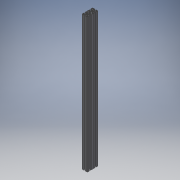
# Autodesk Inventor part: PERFIL_ESTRUTURAL_40X80_EIXO_Y
Saved by Autodesk Inventor 2018 (Build 220112000, 112)
## iProperties
Created: 2018-10-08
Part Number: PERFIL_ESTRUTURAL_40X80_EIXO_Y
Material: Genérico
Document SubType Name: Modeling
Designer: Georgines
Density: 1 g/cm^3
Appearance: Padrão
Author: Georgines
Autodesk Inventor part; units mm, degrees
ref_plane "YZ Plane" through (0, 0, 0) normal (1, 0, 0) x (0, 1, 0)
ref_plane "XZ Plane" through (0, 0, 0) normal (0, 1, 0) x (-1, 0, 0)
ref_plane "XY Plane" through (0, 0, 0) normal (0, 0, 1) x (1, 0, 0)
sketch "Esboço1" plane through (0, 0, 0) normal (0, 0, 1) x (1, 0, 0)
  line L0 (4.1513, 39.5067) -> (4.1513, 35.6766)
  arc A0 (4.3212, 39.6766) -> (4.1513, 39.5067) centre (4.3212, 39.5067) ccw
  line L1 (11.1013, 39.6766) -> (4.3212, 39.6766)
  line L2 (11.1013, 39.4266) -> (11.1013, 39.6766)
  line L3 (13.1013, 39.4266) -> (11.1013, 39.4266)
  line L4 (13.1013, 39.6766) -> (13.1013, 39.4266)
  line L5 (18.6013, 39.6766) -> (13.1013, 39.6766)
  arc A1 (20.1013, 38.1766) -> (18.6013, 39.6766) centre (18.6013, 38.1766) ccw
  line L6 (20.1013, 32.6766) -> (20.1013, 38.1766)
  line L7 (19.8513, 32.6766) -> (20.1013, 32.6766)
  line L8 (19.8513, 30.6766) -> (19.8513, 32.6766)
  line L9 (20.1013, 30.6766) -> (19.8513, 30.6766)
  line L10 (20.1013, 23.8965) -> (20.1013, 30.6766)
  arc A2 (19.9314, 23.7266) -> (20.1013, 23.8965) centre (19.9314, 23.8965) ccw
  line L11 (16.1013, 23.7266) -> (19.9314, 23.7266)
  line L12 (16.1013, 26.8766) -> (16.1013, 23.7266)
  line L13 (18.2013, 26.8766) -> (16.1013, 26.8766)
  line L14 (18.2013, 30.6766) -> (18.2013, 26.8766)
  line L15 (13.6368, 30.6766) -> (18.2013, 30.6766)
  arc A3 (13.6368, 30.6766) -> (12.9297, 30.3837) centre (13.6368, 29.6766) ccw
  line L16 (11.5658, 29.0197) -> (12.9297, 30.3837)
  arc A4 (11.5658, 29.0197) -> (10.1013, 25.4842) centre (15.1013, 25.4842) ccw
  line L17 (10.1013, 13.869) -> (10.1013, 25.4842)
  arc A5 (10.1013, 13.869) -> (11.5658, 10.3334) centre (15.1013, 13.869) ccw
  line L18 (12.9297, 8.9695) -> (11.5658, 10.3334)
  arc A6 (12.9297, 8.9695) -> (13.6368, 8.6766) centre (13.6368, 9.6766) ccw
  line L19 (18.2013, 8.6766) -> (13.6368, 8.6766)
  line L20 (18.2013, 12.4766) -> (18.2013, 8.6766)
  line L21 (16.1013, 12.4766) -> (18.2013, 12.4766)
  line L22 (16.1013, 15.6266) -> (16.1013, 12.4766)
  line L23 (19.9314, 15.6266) -> (16.1013, 15.6266)
  arc A7 (20.1013, 15.4567) -> (19.9314, 15.6266) centre (19.9314, 15.4567) ccw
  line L24 (20.1013, 8.6766) -> (20.1013, 15.4567)
  line L25 (19.8513, 8.6766) -> (20.1013, 8.6766)
  line L26 (19.8513, 6.6766) -> (19.8513, 8.6766)
  line L27 (20.1013, 6.6766) -> (19.8513, 6.6766)
  line L28 (20.1013, -7.3234) -> (20.1013, 6.6766)
  line L29 (19.8513, -7.3234) -> (20.1013, -7.3234)
  line L30 (19.8513, -9.3234) -> (19.8513, -7.3234)
  line L31 (20.1013, -9.3234) -> (19.8513, -9.3234)
  line L32 (20.1013, -16.1035) -> (20.1013, -9.3234)
  arc A8 (19.9314, -16.2734) -> (20.1013, -16.1035) centre (19.9314, -16.1035) ccw
  line L33 (16.1013, -16.2734) -> (19.9314, -16.2734)
  line L34 (16.1013, -13.1234) -> (16.1013, -16.2734)
  line L35 (18.2013, -13.1234) -> (16.1013, -13.1234)
  line L36 (18.2013, -9.3234) -> (18.2013, -13.1234)
  line L37 (13.6368, -9.3234) -> (18.2013, -9.3234)
  arc A9 (13.6368, -9.3234) -> (12.9297, -9.6163) centre (13.6368, -10.3234) ccw
  line L38 (11.5658, -10.9803) -> (12.9297, -9.6163)
  arc A10 (11.5658, -10.9803) -> (10.1013, -14.5158) centre (15.1013, -14.5158) ccw
  line L39 (10.1013, -26.131) -> (10.1013, -14.5158)
  arc A11 (10.1013, -26.131) -> (11.5658, -29.6666) centre (15.1013, -26.131) ccw
  line L40 (12.9297, -31.0305) -> (11.5658, -29.6666)
  arc A12 (12.9297, -31.0305) -> (13.6368, -31.3234) centre (13.6368, -30.3234) ccw
  line L41 (18.2013, -31.3234) -> (13.6368, -31.3234)
  line L42 (18.2013, -27.5234) -> (18.2013, -31.3234)
  line L43 (16.1013, -27.5234) -> (18.2013, -27.5234)
  line L44 (16.1013, -24.3734) -> (16.1013, -27.5234)
  line L45 (19.9314, -24.3734) -> (16.1013, -24.3734)
  arc A13 (20.1013, -24.5433) -> (19.9314, -24.3734) centre (19.9314, -24.5433) ccw
  line L46 (20.1013, -31.3234) -> (20.1013, -24.5433)
  line L47 (19.8513, -31.3234) -> (20.1013, -31.3234)
  line L48 (19.8513, -33.3234) -> (19.8513, -31.3234)
  line L49 (20.1013, -33.3234) -> (19.8513, -33.3234)
  line L50 (20.1013, -38.8234) -> (20.1013, -33.3234)
  arc A14 (18.6013, -40.3234) -> (20.1013, -38.8234) centre (18.6013, -38.8234) ccw
  line L51 (13.1013, -40.3234) -> (18.6013, -40.3234)
  line L52 (13.1013, -40.0734) -> (13.1013, -40.3234)
  line L53 (11.1013, -40.0734) -> (13.1013, -40.0734)
  line L54 (11.1013, -40.3234) -> (11.1013, -40.0734)
  line L55 (4.3212, -40.3234) -> (11.1013, -40.3234)
  arc A15 (4.1513, -40.1535) -> (4.3212, -40.3234) centre (4.3212, -40.1535) ccw
  line L56 (4.1513, -36.3234) -> (4.1513, -40.1535)
  line L57 (7.3013, -36.3234) -> (4.1513, -36.3234)
  line L58 (7.3013, -38.4234) -> (7.3013, -36.3234)
  line L59 (11.1013, -38.4234) -> (7.3013, -38.4234)
  line L60 (11.1013, -33.859) -> (11.1013, -38.4234)
  arc A16 (11.1013, -33.859) -> (10.8084, -33.1519) centre (10.1013, -33.859) ccw
  line L61 (9.4444, -31.7879) -> (10.8084, -33.1519)
  arc A17 (9.4444, -31.7879) -> (5.9089, -30.3234) centre (5.9089, -35.3234) ccw
  line L62 (-5.7063, -30.3234) -> (5.9089, -30.3234)
  arc A18 (-5.7063, -30.3234) -> (-9.2419, -31.7879) centre (-5.7063, -35.3234) ccw
  line L63 (-10.6058, -33.1519) -> (-9.2419, -31.7879)
  arc A19 (-10.6058, -33.1519) -> (-10.8987, -33.859) centre (-9.8987, -33.859) ccw
  line L64 (-10.8987, -38.4234) -> (-10.8987, -33.859)
  line L65 (-7.0987, -38.4234) -> (-10.8987, -38.4234)
  line L66 (-7.0987, -36.3234) -> (-7.0987, -38.4234)
  line L67 (-3.9487, -36.3234) -> (-7.0987, -36.3234)
  line L68 (-3.9487, -40.1535) -> (-3.9487, -36.3234)
  arc A20 (-4.1186, -40.3234) -> (-3.9487, -40.1535) centre (-4.1186, -40.1535) ccw
  line L69 (-10.8987, -40.3234) -> (-4.1186, -40.3234)
  line L70 (-10.8987, -40.0734) -> (-10.8987, -40.3234)
  line L71 (-12.8987, -40.0734) -> (-10.8987, -40.0734)
  line L72 (-12.8987, -40.3234) -> (-12.8987, -40.0734)
  line L73 (-18.3987, -40.3234) -> (-12.8987, -40.3234)
  arc A21 (-19.8987, -38.8234) -> (-18.3987, -40.3234) centre (-18.3987, -38.8234) ccw
  line L74 (-19.8987, -33.3234) -> (-19.8987, -38.8234)
  line L75 (-19.6487, -33.3234) -> (-19.8987, -33.3234)
  line L76 (-19.6487, -31.3234) -> (-19.6487, -33.3234)
  line L77 (-19.8987, -31.3234) -> (-19.6487, -31.3234)
  line L78 (-19.8987, -24.5433) -> (-19.8987, -31.3234)
  arc A22 (-19.7288, -24.3734) -> (-19.8987, -24.5433) centre (-19.7288, -24.5433) ccw
  line L79 (-15.8987, -24.3734) -> (-19.7288, -24.3734)
  line L80 (-15.8987, -27.5234) -> (-15.8987, -24.3734)
  line L81 (-17.9987, -27.5234) -> (-15.8987, -27.5234)
  line L82 (-17.9987, -31.3234) -> (-17.9987, -27.5234)
  line L83 (-13.4342, -31.3234) -> (-17.9987, -31.3234)
  arc A23 (-13.4342, -31.3234) -> (-12.7271, -31.0305) centre (-13.4342, -30.3234) ccw
  line L84 (-11.3632, -29.6666) -> (-12.7271, -31.0305)
  arc A24 (-11.3632, -29.6666) -> (-9.8987, -26.131) centre (-14.8987, -26.131) ccw
  line L85 (-9.8987, -14.5158) -> (-9.8987, -26.131)
  arc A25 (-9.8987, -14.5158) -> (-11.3632, -10.9803) centre (-14.8987, -14.5158) ccw
  line L86 (-12.7271, -9.6163) -> (-11.3632, -10.9803)
  arc A26 (-12.7271, -9.6163) -> (-13.4342, -9.3234) centre (-13.4342, -10.3234) ccw
  line L87 (-17.9987, -9.3234) -> (-13.4342, -9.3234)
  line L88 (-17.9987, -13.1234) -> (-17.9987, -9.3234)
  line L89 (-15.8987, -13.1234) -> (-17.9987, -13.1234)
  line L90 (-15.8987, -16.2734) -> (-15.8987, -13.1234)
  line L91 (-19.7288, -16.2734) -> (-15.8987, -16.2734)
  arc A27 (-19.8987, -16.1035) -> (-19.7288, -16.2734) centre (-19.7288, -16.1035) ccw
  line L92 (-19.8987, -9.3234) -> (-19.8987, -16.1035)
  line L93 (-19.6487, -9.3234) -> (-19.8987, -9.3234)
  line L94 (-19.6487, -7.3234) -> (-19.6487, -9.3234)
  line L95 (-19.8987, -7.3234) -> (-19.6487, -7.3234)
  line L96 (-19.8987, 6.6766) -> (-19.8987, -7.3234)
  line L97 (-19.6487, 6.6766) -> (-19.8987, 6.6766)
  line L98 (-19.6487, 8.6766) -> (-19.6487, 6.6766)
  line L99 (-19.8987, 8.6766) -> (-19.6487, 8.6766)
  line L100 (-19.8987, 15.4567) -> (-19.8987, 8.6766)
  arc A28 (-19.7288, 15.6266) -> (-19.8987, 15.4567) centre (-19.7288, 15.4567) ccw
  line L101 (-15.8987, 15.6266) -> (-19.7288, 15.6266)
  line L102 (-15.8987, 12.4766) -> (-15.8987, 15.6266)
  line L103 (-17.9987, 12.4766) -> (-15.8987, 12.4766)
  line L104 (-17.9987, 8.6766) -> (-17.9987, 12.4766)
  line L105 (-13.4342, 8.6766) -> (-17.9987, 8.6766)
  arc A29 (-13.4342, 8.6766) -> (-12.7271, 8.9695) centre (-13.4342, 9.6766) ccw
  line L106 (-11.3632, 10.3334) -> (-12.7271, 8.9695)
  arc A30 (-11.3632, 10.3334) -> (-9.8987, 13.869) centre (-14.8987, 13.869) ccw
  line L107 (-9.8987, 25.4842) -> (-9.8987, 13.869)
  arc A31 (-9.8987, 25.4842) -> (-11.3632, 29.0197) centre (-14.8987, 25.4842) ccw
  line L108 (-12.7271, 30.3837) -> (-11.3632, 29.0197)
  arc A32 (-12.7271, 30.3837) -> (-13.4342, 30.6766) centre (-13.4342, 29.6766) ccw
  line L109 (-17.9987, 30.6766) -> (-13.4342, 30.6766)
  line L110 (-17.9987, 26.8766) -> (-17.9987, 30.6766)
  line L111 (-15.8987, 26.8766) -> (-17.9987, 26.8766)
  line L112 (-15.8987, 23.7266) -> (-15.8987, 26.8766)
  line L113 (-19.7288, 23.7266) -> (-15.8987, 23.7266)
  arc A33 (-19.8987, 23.8965) -> (-19.7288, 23.7266) centre (-19.7288, 23.8965) ccw
  line L114 (-19.8987, 30.6766) -> (-19.8987, 23.8965)
  line L115 (-19.6487, 30.6766) -> (-19.8987, 30.6766)
  line L116 (-19.6487, 32.6766) -> (-19.6487, 30.6766)
  line L117 (-19.8987, 32.6766) -> (-19.6487, 32.6766)
  line L118 (-19.8987, 38.1766) -> (-19.8987, 32.6766)
  arc A34 (-18.3987, 39.6766) -> (-19.8987, 38.1766) centre (-18.3987, 38.1766) ccw
  line L119 (-12.8987, 39.6766) -> (-18.3987, 39.6766)
  line L120 (-12.8987, 39.4266) -> (-12.8987, 39.6766)
  line L121 (-10.8987, 39.4266) -> (-12.8987, 39.4266)
  line L122 (-10.8987, 39.6766) -> (-10.8987, 39.4266)
  line L123 (-4.1186, 39.6766) -> (-10.8987, 39.6766)
  arc A35 (-3.9487, 39.5067) -> (-4.1186, 39.6766) centre (-4.1186, 39.5067) ccw
  line L124 (-3.9487, 35.6766) -> (-3.9487, 39.5067)
  line L125 (-7.0987, 35.6766) -> (-3.9487, 35.6766)
  line L126 (-7.0987, 37.7766) -> (-7.0987, 35.6766)
  line L127 (-10.8987, 37.7766) -> (-7.0987, 37.7766)
  line L128 (-10.8987, 33.2121) -> (-10.8987, 37.7766)
  arc A36 (-10.8987, 33.2121) -> (-10.6058, 32.505) centre (-9.8987, 33.2121) ccw
  line L129 (-9.2419, 31.141) -> (-10.6058, 32.505)
  arc A37 (-9.2419, 31.141) -> (-5.7063, 29.6766) centre (-5.7063, 34.6766) ccw
  line L130 (5.9089, 29.6766) -> (-5.7063, 29.6766)
  arc A38 (5.9089, 29.6766) -> (9.4444, 31.141) centre (5.9089, 34.6766) ccw
  line L131 (10.8084, 32.505) -> (9.4444, 31.141)
  arc A39 (10.8084, 32.505) -> (11.1013, 33.2121) centre (10.1013, 33.2121) ccw
  line L132 (11.1013, 37.7766) -> (11.1013, 33.2121)
  line L133 (7.3013, 37.7766) -> (11.1013, 37.7766)
  line L134 (7.3013, 35.6766) -> (7.3013, 37.7766)
  line L135 (4.1513, 35.6766) -> (7.3013, 35.6766)
  arc A40 (0.9954, -13.532) -> (-0.7928, -13.532) centre (0.1013, -20.3234) ccw
  line L136 (-0.7928, -13.532) -> (-0.9429, -12.3919)
  arc A41 (-0.9429, -12.3919) -> (-2.9602, -12.9324) centre (0.1013, -20.3234) ccw
  line L137 (-2.9602, -12.9324) -> (-2.5201, -13.9949)
  arc A42 (-2.5201, -13.9949) -> (-3.9834, -14.8245) centre (0.1013, -20.3234) ccw
  line L138 (-3.9834, -14.8245) -> (-4.7102, -14.0977)
  arc A43 (-4.7688, -13.9563) -> (-4.7102, -14.0977) centre (-4.5688, -13.9563) ccw
  line L139 (-4.7688, -13.9563) -> (-4.7688, -12.4524)
  arc A44 (-4.7688, -12.4524) -> (-4.9688, -12.2524) centre (-4.9688, -12.4524) ccw
  line L140 (-4.9688, -12.2524) -> (-7.7698, -12.2524)
  arc A45 (-7.7698, -12.2524) -> (-7.9698, -12.4524) centre (-7.7698, -12.4524) ccw
  line L141 (-7.9698, -12.4524) -> (-7.9698, -15.2533)
  arc A46 (-7.9698, -15.2533) -> (-7.7698, -15.4533) centre (-7.7698, -15.2533) ccw
  line L142 (-7.7698, -15.4533) -> (-6.2659, -15.4533)
  arc A47 (-6.1244, -15.5119) -> (-6.2659, -15.4533) centre (-6.2659, -15.6533) ccw
  line L143 (-6.1244, -15.5119) -> (-5.3976, -16.2388)
  arc A48 (-5.3976, -16.2388) -> (-6.2273, -17.7021) centre (0.1013, -20.3234) ccw
  line L144 (-6.2273, -17.7021) -> (-7.2897, -17.262)
  arc A49 (-7.2897, -17.262) -> (-7.8303, -19.2792) centre (0.1013, -20.3234) ccw
  line L145 (-7.8303, -19.2792) -> (-6.6901, -19.4293)
  arc A50 (-6.6901, -19.4293) -> (-6.6901, -21.2175) centre (0.1013, -20.3234) ccw
  line L146 (-6.6901, -21.2175) -> (-7.8303, -21.3676)
  arc A51 (-7.8303, -21.3676) -> (-7.2897, -23.3849) centre (0.1013, -20.3234) ccw
  line L147 (-7.2897, -23.3849) -> (-6.2273, -22.9448)
  arc A52 (-6.2273, -22.9448) -> (-5.3976, -24.4081) centre (0.1013, -20.3234) ccw
  line L148 (-5.3976, -24.4081) -> (-6.1244, -25.1349)
  arc A53 (-6.2659, -25.1935) -> (-6.1244, -25.1349) centre (-6.2659, -24.9935) ccw
  line L149 (-6.2659, -25.1935) -> (-7.7698, -25.1935)
  arc A54 (-7.7698, -25.1935) -> (-7.9698, -25.3935) centre (-7.7698, -25.3935) ccw
  line L150 (-7.9698, -25.3935) -> (-7.9698, -28.1945)
  arc A55 (-7.9698, -28.1945) -> (-7.7698, -28.3945) centre (-7.7698, -28.1945) ccw
  line L151 (-7.7698, -28.3945) -> (-4.9688, -28.3945)
  arc A56 (-4.9688, -28.3945) -> (-4.7688, -28.1945) centre (-4.9688, -28.1945) ccw
  line L152 (-4.7688, -28.1945) -> (-4.7688, -26.6906)
  arc A57 (-4.7102, -26.5492) -> (-4.7688, -26.6906) centre (-4.5688, -26.6906) ccw
  line L153 (-4.7102, -26.5492) -> (-3.9834, -25.8223)
  arc A58 (-3.9834, -25.8223) -> (-2.5201, -26.652) centre (0.1013, -20.3234) ccw
  line L154 (-2.5201, -26.652) -> (-2.9602, -27.7145)
  arc A59 (-2.9602, -27.7145) -> (-0.9429, -28.255) centre (0.1013, -20.3234) ccw
  line L155 (-0.9429, -28.255) -> (-0.7928, -27.1148)
  arc A60 (-0.7928, -27.1148) -> (0.9954, -27.1148) centre (0.1013, -20.3234) ccw
  line L156 (0.9954, -27.1148) -> (1.1455, -28.255)
  arc A61 (1.1455, -28.255) -> (3.1628, -27.7145) centre (0.1013, -20.3234) ccw
  line L157 (3.1628, -27.7145) -> (2.7227, -26.652)
  arc A62 (2.7227, -26.652) -> (4.186, -25.8223) centre (0.1013, -20.3234) ccw
  line L158 (4.186, -25.8223) -> (4.9128, -26.5492)
  arc A63 (4.9714, -26.6906) -> (4.9128, -26.5492) centre (4.7714, -26.6906) ccw
  line L159 (4.9714, -26.6906) -> (4.9714, -28.1945)
  arc A64 (4.9714, -28.1945) -> (5.1714, -28.3945) centre (5.1714, -28.1945) ccw
  line L160 (5.1714, -28.3945) -> (7.9724, -28.3945)
  arc A65 (7.9724, -28.3945) -> (8.1724, -28.1945) centre (7.9724, -28.1945) ccw
  line L161 (8.1724, -28.1945) -> (8.1724, -25.3935)
  arc A66 (8.1724, -25.3935) -> (7.9724, -25.1935) centre (7.9724, -25.3935) ccw
  line L162 (7.9724, -25.1935) -> (6.4684, -25.1935)
  arc A67 (6.327, -25.1349) -> (6.4684, -25.1935) centre (6.4684, -24.9935) ccw
  line L163 (6.327, -25.1349) -> (5.6002, -24.4081)
  arc A68 (5.6002, -24.4081) -> (6.4299, -22.9448) centre (0.1013, -20.3234) ccw
  line L164 (6.4299, -22.9448) -> (7.4923, -23.3849)
  arc A69 (7.4923, -23.3849) -> (8.0328, -21.3676) centre (0.1013, -20.3234) ccw
  line L165 (8.0328, -21.3676) -> (6.8927, -21.2175)
  arc A70 (6.8927, -21.2175) -> (6.8927, -19.4293) centre (0.1013, -20.3234) ccw
  line L166 (6.8927, -19.4293) -> (8.0328, -19.2792)
  arc A71 (8.0328, -19.2792) -> (7.4923, -17.262) centre (0.1013, -20.3234) ccw
  line L167 (7.4923, -17.262) -> (6.4299, -17.7021)
  arc A72 (6.4299, -17.7021) -> (5.6002, -16.2388) centre (0.1013, -20.3234) ccw
  line L168 (5.6002, -16.2388) -> (6.327, -15.5119)
  arc A73 (6.4684, -15.4533) -> (6.327, -15.5119) centre (6.4684, -15.6533) ccw
  line L169 (6.4684, -15.4533) -> (7.9724, -15.4533)
  arc A74 (7.9724, -15.4533) -> (8.1724, -15.2533) centre (7.9724, -15.2533) ccw
  line L170 (8.1724, -15.2533) -> (8.1724, -12.4524)
  arc A75 (8.1724, -12.4524) -> (7.9724, -12.2524) centre (7.9724, -12.4524) ccw
  line L171 (7.9724, -12.2524) -> (5.1714, -12.2524)
  arc A76 (5.1714, -12.2524) -> (4.9714, -12.4524) centre (5.1714, -12.4524) ccw
  line L172 (4.9714, -12.4524) -> (4.9714, -13.9563)
  arc A77 (4.9128, -14.0977) -> (4.9714, -13.9563) centre (4.7714, -13.9563) ccw
  line L173 (4.9128, -14.0977) -> (4.186, -14.8245)
  arc A78 (4.186, -14.8245) -> (2.7227, -13.9949) centre (0.1013, -20.3234) ccw
  line L174 (2.7227, -13.9949) -> (3.1628, -12.9324)
  arc A79 (3.1628, -12.9324) -> (1.1455, -12.3919) centre (0.1013, -20.3234) ccw
  line L175 (1.1455, -12.3919) -> (0.9954, -13.532)
  arc A80 (-14.2427, -33.6068) -> (-16.5547, -33.6068) centre (-15.3987, -35.8234) ccw
  line L176 (-16.5547, -33.6068) -> (-16.8129, -33.3486)
  arc A81 (-16.8129, -33.3486) -> (-17.8736, -34.4092) centre (-17.3433, -33.8789) ccw
  line L177 (-17.8736, -34.4092) -> (-17.6154, -34.6674)
  arc A82 (-17.6154, -34.6674) -> (-17.6154, -36.9794) centre (-15.3987, -35.8234) ccw
  line L178 (-17.6154, -36.9794) -> (-17.8736, -37.2376)
  arc A83 (-17.8736, -37.2376) -> (-16.8129, -38.2983) centre (-17.3433, -37.768) ccw
  line L179 (-16.8129, -38.2983) -> (-16.5547, -38.0401)
  arc A84 (-16.5547, -38.0401) -> (-14.2427, -38.0401) centre (-15.3987, -35.8234) ccw
  line L180 (-14.2427, -38.0401) -> (-13.9845, -38.2983)
  arc A85 (-13.9845, -38.2983) -> (-12.9238, -37.2376) centre (-13.4542, -37.768) ccw
  line L181 (-12.9238, -37.2376) -> (-13.182, -36.9794)
  arc A86 (-13.182, -36.9794) -> (-13.182, -34.6674) centre (-15.3987, -35.8234) ccw
  line L182 (-13.182, -34.6674) -> (-12.9238, -34.4092)
  arc A87 (-12.9238, -34.4092) -> (-13.9845, -33.3486) centre (-13.4542, -33.8789) ccw
  line L183 (-13.9845, -33.3486) -> (-14.2427, -33.6068)
  arc A88 (14.4453, 32.9599) -> (16.7573, 32.9599) centre (15.6013, 35.1766) ccw
  line L184 (16.7573, 32.9599) -> (17.0155, 32.7017)
  arc A89 (17.0155, 32.7017) -> (18.0762, 33.7624) centre (17.5458, 33.232) ccw
  line L185 (18.0762, 33.7624) -> (17.818, 34.0206)
  arc A90 (17.818, 34.0206) -> (17.818, 36.3326) centre (15.6013, 35.1766) ccw
  line L186 (17.818, 36.3326) -> (18.0762, 36.5908)
  arc A91 (18.0762, 36.5908) -> (17.0155, 37.6514) centre (17.5458, 37.1211) ccw
  line L187 (17.0155, 37.6514) -> (16.7573, 37.3932)
  arc A92 (16.7573, 37.3932) -> (14.4453, 37.3932) centre (15.6013, 35.1766) ccw
  line L188 (14.4453, 37.3932) -> (14.1871, 37.6514)
  arc A93 (14.1871, 37.6514) -> (13.1264, 36.5908) centre (13.6567, 37.1211) ccw
  line L189 (13.1264, 36.5908) -> (13.3846, 36.3326)
  arc A94 (13.3846, 36.3326) -> (13.3846, 34.0206) centre (15.6013, 35.1766) ccw
  line L190 (13.3846, 34.0206) -> (13.1264, 33.7624)
  arc A95 (13.1264, 33.7624) -> (14.1871, 32.7017) centre (13.6567, 33.232) ccw
  line L191 (14.1871, 32.7017) -> (14.4453, 32.9599)
  arc A96 (-17.6154, 36.3326) -> (-17.6154, 34.0206) centre (-15.3987, 35.1766) ccw
  line L192 (-17.6154, 34.0206) -> (-17.8736, 33.7624)
  arc A97 (-17.8736, 33.7624) -> (-16.8129, 32.7017) centre (-17.3433, 33.232) ccw
  line L193 (-16.8129, 32.7017) -> (-16.5547, 32.9599)
  arc A98 (-16.5547, 32.9599) -> (-14.2427, 32.9599) centre (-15.3987, 35.1766) ccw
  line L194 (-14.2427, 32.9599) -> (-13.9845, 32.7017)
  arc A99 (-13.9845, 32.7017) -> (-12.9238, 33.7624) centre (-13.4542, 33.232) ccw
  line L195 (-12.9238, 33.7624) -> (-13.182, 34.0206)
  arc A100 (-13.182, 34.0206) -> (-13.182, 36.3326) centre (-15.3987, 35.1766) ccw
  line L196 (-13.182, 36.3326) -> (-12.9238, 36.5908)
  arc A101 (-12.9238, 36.5908) -> (-13.9845, 37.6514) centre (-13.4542, 37.1211) ccw
  line L197 (-13.9845, 37.6514) -> (-14.2427, 37.3932)
  arc A102 (-14.2427, 37.3932) -> (-16.5547, 37.3932) centre (-15.3987, 35.1766) ccw
  line L198 (-16.5547, 37.3932) -> (-16.8129, 37.6514)
  arc A103 (-16.8129, 37.6514) -> (-17.8736, 36.5908) centre (-17.3433, 37.1211) ccw
  line L199 (-17.8736, 36.5908) -> (-17.6154, 36.3326)
  arc A104 (14.4453, -38.0401) -> (16.7573, -38.0401) centre (15.6013, -35.8234) ccw
  line L200 (16.7573, -38.0401) -> (17.0155, -38.2983)
  arc A105 (17.0155, -38.2983) -> (18.0762, -37.2376) centre (17.5458, -37.768) ccw
  line L201 (18.0762, -37.2376) -> (17.818, -36.9794)
  arc A106 (17.818, -36.9794) -> (17.818, -34.6674) centre (15.6013, -35.8234) ccw
  line L202 (17.818, -34.6674) -> (18.0762, -34.4092)
  arc A107 (18.0762, -34.4092) -> (17.0155, -33.3486) centre (17.5458, -33.8789) ccw
  line L203 (17.0155, -33.3486) -> (16.7573, -33.6068)
  arc A108 (16.7573, -33.6068) -> (14.4453, -33.6068) centre (15.6013, -35.8234) ccw
  line L204 (14.4453, -33.6068) -> (14.1871, -33.3486)
  arc A109 (14.1871, -33.3486) -> (13.1264, -34.4092) centre (13.6567, -33.8789) ccw
  line L205 (13.1264, -34.4092) -> (13.3846, -34.6674)
  arc A110 (13.3846, -34.6674) -> (13.3846, -36.9794) centre (15.6013, -35.8234) ccw
  line L206 (13.3846, -36.9794) -> (13.1264, -37.2376)
  arc A111 (13.1264, -37.2376) -> (14.1871, -38.2983) centre (13.6567, -37.768) ccw
  line L207 (14.1871, -38.2983) -> (14.4453, -38.0401)
  arc A112 (6.4684, 24.5467) -> (6.327, 24.4881) centre (6.4684, 24.3467) ccw
  line L208 (6.4684, 24.5467) -> (7.9724, 24.5467)
  arc A113 (7.9724, 24.5467) -> (8.1724, 24.7467) centre (7.9724, 24.7467) ccw
  line L209 (8.1724, 24.7467) -> (8.1724, 27.5476)
  arc A114 (8.1724, 27.5476) -> (7.9724, 27.7476) centre (7.9724, 27.5476) ccw
  line L210 (7.9724, 27.7476) -> (5.1714, 27.7476)
  arc A115 (5.1714, 27.7476) -> (4.9714, 27.5476) centre (5.1714, 27.5476) ccw
  line L211 (4.9714, 27.5476) -> (4.9714, 26.0437)
  arc A116 (4.9128, 25.9023) -> (4.9714, 26.0437) centre (4.7714, 26.0437) ccw
  line L212 (4.9128, 25.9023) -> (4.186, 25.1755)
  arc A117 (4.186, 25.1755) -> (2.7227, 26.0051) centre (0.1013, 19.6766) ccw
  line L213 (2.7227, 26.0051) -> (3.1628, 27.0676)
  arc A118 (3.1628, 27.0676) -> (1.1455, 27.6081) centre (0.1013, 19.6766) ccw
  line L214 (1.1455, 27.6081) -> (0.9954, 26.468)
  arc A119 (0.9954, 26.468) -> (-0.7928, 26.468) centre (0.1013, 19.6766) ccw
  line L215 (-0.7928, 26.468) -> (-0.9429, 27.6081)
  arc A120 (-0.9429, 27.6081) -> (-2.9602, 27.0676) centre (0.1013, 19.6766) ccw
  line L216 (-2.9602, 27.0676) -> (-2.5201, 26.0051)
  arc A121 (-2.5201, 26.0051) -> (-3.9834, 25.1755) centre (0.1013, 19.6766) ccw
  line L217 (-3.9834, 25.1755) -> (-4.7102, 25.9023)
  arc A122 (-4.7688, 26.0437) -> (-4.7102, 25.9023) centre (-4.5688, 26.0437) ccw
  line L218 (-4.7688, 26.0437) -> (-4.7688, 27.5476)
  arc A123 (-4.7688, 27.5476) -> (-4.9688, 27.7476) centre (-4.9688, 27.5476) ccw
  line L219 (-4.9688, 27.7476) -> (-7.7698, 27.7476)
  arc A124 (-7.7698, 27.7476) -> (-7.9698, 27.5476) centre (-7.7698, 27.5476) ccw
  line L220 (-7.9698, 27.5476) -> (-7.9698, 24.7467)
  arc A125 (-7.9698, 24.7467) -> (-7.7698, 24.5467) centre (-7.7698, 24.7467) ccw
  line L221 (-7.7698, 24.5467) -> (-6.2659, 24.5467)
  arc A126 (-6.1244, 24.4881) -> (-6.2659, 24.5467) centre (-6.2659, 24.3467) ccw
  line L222 (-6.1244, 24.4881) -> (-5.3976, 23.7612)
  arc A127 (-5.3976, 23.7612) -> (-6.2273, 22.2979) centre (0.1013, 19.6766) ccw
  line L223 (-6.2273, 22.2979) -> (-7.2897, 22.738)
  arc A128 (-7.2897, 22.738) -> (-7.8303, 20.7208) centre (0.1013, 19.6766) ccw
  line L224 (-7.8303, 20.7208) -> (-6.6901, 20.5707)
  arc A129 (-6.6901, 20.5707) -> (-6.6901, 18.7825) centre (0.1013, 19.6766) ccw
  line L225 (-6.6901, 18.7825) -> (-7.8303, 18.6324)
  arc A130 (-7.8303, 18.6324) -> (-7.2897, 16.6151) centre (0.1013, 19.6766) ccw
  line L226 (-7.2897, 16.6151) -> (-6.2273, 17.0552)
  arc A131 (-6.2273, 17.0552) -> (-5.3976, 15.5919) centre (0.1013, 19.6766) ccw
  line L227 (-5.3976, 15.5919) -> (-6.1244, 14.8651)
  arc A132 (-6.2659, 14.8065) -> (-6.1244, 14.8651) centre (-6.2659, 15.0065) ccw
  line L228 (-6.2659, 14.8065) -> (-7.7698, 14.8065)
  arc A133 (-7.7698, 14.8065) -> (-7.9698, 14.6065) centre (-7.7698, 14.6065) ccw
  line L229 (-7.9698, 14.6065) -> (-7.9698, 11.8055)
  arc A134 (-7.9698, 11.8055) -> (-7.7698, 11.6055) centre (-7.7698, 11.8055) ccw
  line L230 (-7.7698, 11.6055) -> (-4.9688, 11.6055)
  arc A135 (-4.9688, 11.6055) -> (-4.7688, 11.8055) centre (-4.9688, 11.8055) ccw
  line L231 (-4.7688, 11.8055) -> (-4.7688, 13.3094)
  arc A136 (-4.7102, 13.4508) -> (-4.7688, 13.3094) centre (-4.5688, 13.3094) ccw
  line L232 (-4.7102, 13.4508) -> (-3.9834, 14.1777)
  arc A137 (-3.9834, 14.1777) -> (-2.5201, 13.348) centre (0.1013, 19.6766) ccw
  line L233 (-2.5201, 13.348) -> (-2.9602, 12.2855)
  arc A138 (-2.9602, 12.2855) -> (-0.9429, 11.745) centre (0.1013, 19.6766) ccw
  line L234 (-0.9429, 11.745) -> (-0.7928, 12.8852)
  arc A139 (-0.7928, 12.8852) -> (0.9954, 12.8852) centre (0.1013, 19.6766) ccw
  line L235 (0.9954, 12.8852) -> (1.1455, 11.745)
  arc A140 (1.1455, 11.745) -> (3.1628, 12.2855) centre (0.1013, 19.6766) ccw
  line L236 (3.1628, 12.2855) -> (2.7227, 13.348)
  arc A141 (2.7227, 13.348) -> (4.186, 14.1777) centre (0.1013, 19.6766) ccw
  line L237 (4.186, 14.1777) -> (4.9128, 13.4508)
  arc A142 (4.9714, 13.3094) -> (4.9128, 13.4508) centre (4.7714, 13.3094) ccw
  line L238 (4.9714, 13.3094) -> (4.9714, 11.8055)
  arc A143 (4.9714, 11.8055) -> (5.1714, 11.6055) centre (5.1714, 11.8055) ccw
  line L239 (5.1714, 11.6055) -> (7.9724, 11.6055)
  arc A144 (7.9724, 11.6055) -> (8.1724, 11.8055) centre (7.9724, 11.8055) ccw
  line L240 (8.1724, 11.8055) -> (8.1724, 14.6065)
  arc A145 (8.1724, 14.6065) -> (7.9724, 14.8065) centre (7.9724, 14.6065) ccw
  line L241 (7.9724, 14.8065) -> (6.4684, 14.8065)
  arc A146 (6.327, 14.8651) -> (6.4684, 14.8065) centre (6.4684, 15.0065) ccw
  line L242 (6.327, 14.8651) -> (5.6002, 15.5919)
  arc A147 (5.6002, 15.5919) -> (6.4299, 17.0552) centre (0.1013, 19.6766) ccw
  line L243 (6.4299, 17.0552) -> (7.4923, 16.6151)
  arc A148 (7.4923, 16.6151) -> (8.0328, 18.6324) centre (0.1013, 19.6766) ccw
  line L244 (8.0328, 18.6324) -> (6.8927, 18.7825)
  arc A149 (6.8927, 18.7825) -> (6.8927, 20.5707) centre (0.1013, 19.6766) ccw
  line L245 (6.8927, 20.5707) -> (8.0328, 20.7208)
  arc A150 (8.0328, 20.7208) -> (7.4923, 22.738) centre (0.1013, 19.6766) ccw
  line L246 (7.4923, 22.738) -> (6.4299, 22.2979)
  arc A151 (6.4299, 22.2979) -> (5.6002, 23.7612) centre (0.1013, 19.6766) ccw
  line L247 (5.6002, 23.7612) -> (6.327, 24.4881)
  line L248 (-9.4907, 8.7409) -> (-11.0152, 7.2164)
  line L249 (-11.0152, 7.2164) -> (-13.2909, 6)
  line L250 (-13.2909, 6) -> (-18, 6)
  line L251 (-18, 6) -> (-18, -6)
  line L252 (-18, -6) -> (-13.2909, -6)
  line L253 (-13.2909, -6) -> (-11.0152, -7.2164)
  line L254 (-11.0152, -7.2164) -> (-9.4907, -8.7409)
  arc A152 (-9.4907, -8.7409) -> (-5.9552, -10.2054) centre (-5.9552, -5.2054) ccw
  line L255 (-5.9552, -10.2054) -> (5.9552, -10.2054)
  arc A153 (5.9552, -10.2054) -> (9.4907, -8.7409) centre (5.9552, -5.2054) ccw
  line L256 (9.4907, -8.7409) -> (11.0152, -7.2164)
  line L257 (11.0152, -7.2164) -> (13.2909, -6)
  line L258 (13.2909, -6) -> (18, -6)
  line L259 (18, -6) -> (18, 6)
  line L260 (18, 6) -> (13.2909, 6)
  line L261 (13.2909, 6) -> (11.0152, 7.2164)
  line L262 (11.0152, 7.2164) -> (9.4907, 8.7409)
  arc A154 (9.4907, 8.7409) -> (5.9552, 10.2054) centre (5.9552, 5.2054) ccw
  line L263 (5.9552, 10.2054) -> (-5.9552, 10.2054)
  arc A155 (-5.9552, 10.2054) -> (-9.4907, 8.7409) centre (-5.9552, 5.2054) ccw
  line L264 (-18, 0) -> (18, 0) construction
  line L265 (0, 10.2054) -> (0, -10.2054) construction
  point P0 (0, 0)
  point P1 (20.1013, -0.3234)
  point P2 (0, 0)
  constraints: 532 end point, 312 point on circle, 156 centre point, 5 midpoint, 1 coincident
extrude "Extrusão1" add sketch "Esboço1" along normal blind 1000
